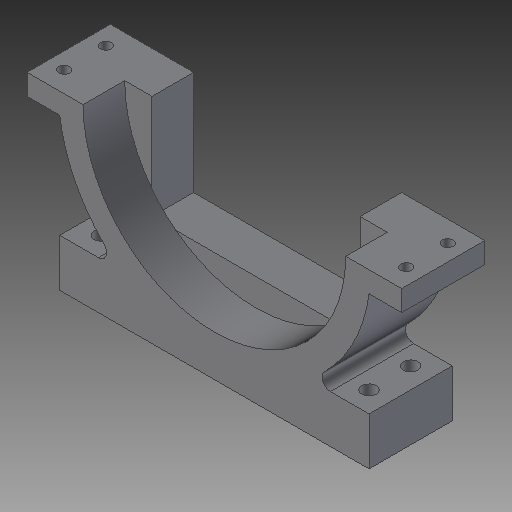
# Autodesk Inventor part: 2124_Bearing Clamps NoPulley_V2
Saved by Autodesk Inventor 2020 (Build 240168000, 168)
## iProperties
Created: 2017-06-21
Part Number: 2124_Bearing Clamps NoPulley_V2
Material: ABS Plastic
Document SubType Name: Modeling
Designer: MPI
Density: 1.06 g/cm^3
Appearance: Smooth - White
Mass: 514.652 g
Surface Area: 684.25 cm^2
Volume: 485.521 cm^3
Author: MPI
Autodesk Inventor part; units mm, degrees
ref_plane "YZ Plane" through (0, 0, 0) normal (1, 0, 0) x (0, 1, 0)
ref_plane "XZ Plane" through (0, 0, 0) normal (0, 1, 0) x (-1, 0, 0)
ref_plane "XY Plane" through (0, 0, 0) normal (0, 0, 1) x (1, 0, 0)
sketch "Sketch1" plane through (0, 0, 0) normal (0, 0, 1) x (1, 0, 0)
  circle A0 centre (0, 0) radius 80.137
  line L0 (-114.3, -12.7) -> (-114.3, 12.7)
  line L1 (114.3, 12.7) -> (114.3, -12.7)
  line L2 (114.3, -12.7) -> (-114.3, 12.7) construction
  line L3 (-114.3, -12.7) -> (114.3, 12.7) construction
  line L4 (-114.3, 0) -> (95.25, 0) construction
  line L5 (-114.3, 12.7) -> (-94.3995, 12.7)
  line L6 (94.3995, 12.7) -> (114.3, 12.7)
  arc A1 (-94.3995, -12.7) -> (94.3995, -12.7) centre (0, 0) ccw
  arc A2 (94.3995, 12.7) -> (-94.3995, 12.7) centre (0, 0) ccw
  line L7 (114.3, -12.7) -> (94.3995, -12.7)
  line L8 (-94.3995, -12.7) -> (-114.3, -12.7)
  dimension "d0" = 160.274
  dimension "d2" = 228.6
  dimension "d3" = 25.4
  constraints: 18 end point, 7 parallel, 4 point on circle, 3 centre point, 3 midpoint, 2 coincident, 2 horizontal, 2 perpendicular
  measures "d0" diameter of A0
  measures "d2" distance of L1.end L0.start
  measures "d3" distance of L0.start L0.end
extrude "Extrusion1" add sketch "Sketch1" along normal blind 25.4
sketch "Sketch2" plane through (94.3995, 12.7, 0) normal (0, 1, 0) x (1, 0, 0)
  line L0 (19.9005, 0) -> (0, 0) projected
  line L1 (0, 0) -> (0, -25.4) projected
  line L2 (19.9005, -25.4) -> (0, -25.4) projected
  line L3 (19.9005, 0) -> (19.9005, -25.4) projected
  line L4 (19.9005, -12.7) -> (0, -12.7) construction
  line L5 (9.9502, -25.4) -> (9.9502, 0) construction
  circle A0 centre (9.9502, -12.7) radius 3.3782
  point P0 (-94.3995, 0)
  dimension "d6" = 6.7564
  constraints: 5 midpoint, 4 end point, 1 centre point
  measures "d6" diameter of A0
extrude "Extrusion2" cut sketch "Sketch2" against normal blind 38.1 contours A0
sketch "Sketch3" plane through (94.3995, 12.7, 0) normal (0, 1, 0) x (1, 0, 0)
  circle A0 centre (9.9502, -12.7) radius 3.175
  line L0 (9.9502, -4.8005) -> (16.7914, -8.7502)
  line L1 (16.7914, -8.7502) -> (16.7914, -16.6498)
  line L2 (16.7914, -16.6498) -> (9.9502, -20.5995)
  line L3 (9.9502, -20.5995) -> (3.1091, -16.6498)
  line L4 (3.1091, -16.6498) -> (3.1091, -8.7502)
  line L5 (3.1091, -8.7502) -> (9.9502, -4.8005)
  point P0 (-94.3995, 0)
  constraints: 12 end point, 1 centre point, 1 coincident, 13 other
extrude "Extrusion3" [suppressed]
mirror "Mirror1" about plane through (0, 0, 0) normal (1, 0, 0) of "Extrusion2"
sketch "Sketch6" plane through (0, 0, 25.4) normal (0, 0, 1) x (1, 0, 0)
  line L0 (-63.5, -63.5) -> (-63.5, 63.5) construction
  line L1 (-63.5, 63.5) -> (63.5, 63.5) construction
  line L2 (63.5, 63.5) -> (63.5, -63.5) construction
  line L3 (63.5, -63.5) -> (-63.5, -63.5) construction
  line L4 (-94.3995, 94.3995) -> (-63.5, 63.5) construction
  line L5 (63.5, 63.5) -> (94.3995, 94.3995) construction
  line L6 (63.5, -63.5) -> (94.3995, -94.3995) construction
  line L7 (-63.5, -63.5) -> (63.5, -63.5) construction
  line L8 (-63.5, -63.5) -> (-94.3995, -94.3995) construction
  point P0 (-78.9498, 78.9498)
  point P1 (78.9498, 78.9498)
  point P2 (78.9498, -78.9498)
  point P3 (-78.9498, -78.9498)
  constraints: 8 end point, 4 midpoint, 3 perpendicular
hole "Hole1" [suppressed]
sketch "Sketch9" plane through (0, 0, 25.4) normal (0, 0, 1) x (1, 0, 0)
  line L0 (114.3, -12.7) -> (114.3, 12.7) projected
  line L1 (114.3, 12.7) -> (94.3995, 12.7) projected
  line L2 (94.3995, 12.7) -> (94.3995, 94.3995) projected
  line L3 (94.3995, 94.3995) -> (12.7, 94.3995) projected
  arc A0 (94.3995, 12.7) -> (-94.3995, 12.7) centre (0, 0) ccw projected
  line L4 (-12.7, 94.3995) -> (-94.3995, 94.3995) projected
  line L5 (-94.3995, 94.3995) -> (-94.3995, 12.7) projected
  line L6 (-94.3995, 12.7) -> (-114.3, 12.7) projected
  line L7 (-114.3, 12.7) -> (-114.3, -12.7) projected
  line L8 (-114.3, 0) -> (114.3, 0)
  constraints: 2 end point, 2 midpoint
extrude "Extrusion7" cut sketch "Sketch9" against normal blind 25.4
sketch "Sketch10" plane through (0, 0, 0) normal (0, 0, -1) x (-1, 0, 0)
  arc A0 (-94.3995, -12.7) -> (94.3995, -12.7) centre (0, 0) ccw projected
  line L0 (-63.5, -63.5) -> (63.5, -63.5)
  line L1 (63.5, -63.5) -> (63.5, 63.5)
  line L2 (63.5, 63.5) -> (-63.5, 63.5)
  line L3 (-63.5, 63.5) -> (-63.5, -63.5)
  line L4 (-63.5, -63.5) -> (63.5, 63.5) construction
  line L5 (63.5, -63.5) -> (-63.5, 63.5) construction
  circle A1 centre (0, 0) radius 95.25
  dimension "d58" = 127
  dimension "d59" = 127
  constraints: 12 end point, 2 midpoint, 2 parallel, 1 centre point, 1 coincident, 1 horizontal, 1 perpendicular
  measures "d58" distance of L2.end L1.end
  measures "d59" distance of L1.end L0.end
extrude "Extrusion8" add sketch "Sketch10" along normal blind 25.4
sketch "Sketch12" plane through (0, 0, 0) normal (0, 0, 1) x (1, 0, 0)
  line L0 (-80.137, 0) -> (-114.3, 0) projected
  line L1 (-114.3, 0) -> (111.125, 0)
  line L2 (111.125, 0) -> (111.125, 104.775)
  line L3 (111.125, 104.775) -> (-114.3, 104.775)
  line L4 (-114.3, 104.775) -> (-114.3, 0)
  point P0 (0, 0)
  point P1 (-83.312, 0)
  constraints: 8 end point, 2 parallel, 1 horizontal, 1 perpendicular
extrude "Extrusion10" cut sketch "Sketch12" against normal blind 25.4
sketch "Sketch14" plane through (0, 0, 25.4) normal (0, 0, 1) x (1, 0, 0)
  line L0 (80.137, 0) -> (63.5, 0) projected
  line L1 (-114.3, -12.7) -> (-94.3995, -12.7) projected
  line L2 (94.3995, -105.25) -> (-94.3995, -105.25)
  line L3 (0, -95.25) -> (-39.6875, -95.25)
  arc A0 (-94.3995, -12.7) -> (94.3995, -12.7) centre (0, 0) ccw
  line L4 (94.3995, -76.2) -> (57.15, -76.2)
  line L5 (-94.3995, -76.2) -> (-57.15, -76.2)
  arc A1 (-57.15, -76.2) -> (57.15, -76.2) centre (0, 0) ccw
  line L6 (94.3995, -105.25) -> (94.3995, -76.2)
  line L7 (-94.3995, -105.25) -> (-94.3995, -76.2)
  point P0 (-80.137, 0)
  dimension "d74" = 10
  constraints: 12 end point, 6 point on circle, 2 centre point, 2 coincident, 2 horizontal, 2 point on line, 1 parallel, 1 vertical
  measures "d74" distance between parallel lines of L2 L3
extrude "Extrusion11" add sketch "Sketch14" against normal up to surface (50.8 mm away)
fillet "Fillet1" radius 5.08 4 edges at (-57.15, -76.2, 12.7) (-57.15, -76.2, -12.7) (57.15, -76.2, 12.7) (57.15, -76.2, -12.7)
sketch "Sketch16" plane through (-94.3995, -105.25, 25.4) normal (0, -1, 0) x (1, 0, 0)
  circle A0 centre (12.7, -38.1) radius 4.5
  line L0 (0, 0) -> (0, -50.8) projected
  line L1 (188.7991, -50.8) -> (0, -50.8) projected
  circle A1 centre (12.7, -12.7) radius 4.5
  line L2 (0, 0) -> (188.7991, 0) projected
  circle A2 centre (176.0991, -38.1) radius 4.5
  circle A3 centre (176.0991, -12.7) radius 4.5
  line L3 (188.7991, 0) -> (188.7991, -50.8) projected
  point P0 (94.3995, -25.4)
  dimension "d76" = 9
  dimension "d77" = 12.7
  dimension "d78" = 12.7
  dimension "d79" = 9
  dimension "d80" = 12.7
  dimension "d81" = 12.7
  dimension "d82" = 9
  dimension "d83" = 9
  dimension "d84" = 12.7
  dimension "d85" = 12.7
  dimension "d88" = 12.7
  dimension "d89" = 12.7
  constraints: 4 centre point
  measures "d76" diameter of A0
  measures "d77" distance from line of L0 A0.centre
  measures "d78" distance from line of L1 A0.centre
  measures "d79" diameter of A1
  measures "d80" distance from line of L0 A1.centre
  measures "d81" distance from line of L2 A1.centre
  measures "d82" diameter of A2
  measures "d83" diameter of A3
  measures "d84" distance from line of L3 A2.centre
  measures "d85" distance from line of L3 A3.centre
  measures "d88" distance from line of L1 A2.centre
  measures "d89" distance from line of L2 A3.centre
extrude "Extrusion12" cut sketch "Sketch16" against normal up to surface (29.05 mm away) contours A0 | A1 | A2 | A3
sketch "Sketch17" plane through (0, 0, 0) normal (0, 0, -1) x (-1, 0, 0)
  arc A0 (-95.25, 0) -> (-94.3995, -12.7) centre (0, 0) ccw projected
  line L0 (-95.25, 0) -> (-114.3, 0) projected
  line L1 (-114.3, -12.7) -> (-114.3, 0) projected
  line L2 (-94.3995, -12.7) -> (-114.3, -12.7) projected
  arc A1 (94.3995, -12.7) -> (95.25, 0) centre (0, 0) ccw projected
  line L3 (114.3, -12.7) -> (94.3995, -12.7) projected
  line L4 (114.3, 0) -> (114.3, -12.7) projected
  line L5 (114.3, 0) -> (95.25, 0) projected
extrude "Extrusion13" add sketch "Sketch17" along normal blind 25.4
sketch "Sketch18" plane through (-114.3, -12.7, 25.4) normal (0, -1, 0) x (1, 0, 0)
  circle A0 centre (9.9502, -12.7) radius 3.3782 projected
  circle A1 centre (9.9502, -38.1) radius 3.3782
  line L0 (0, 0) -> (19.9005, 0) projected
  line L1 (19.9005, -50.8) -> (0, -50.8) projected
  line L2 (0, -50.8) -> (0, 0) projected
  circle A2 centre (218.6498, -12.7) radius 3.3782 projected
  circle A3 centre (218.6498, -38.1) radius 3.3782
  line L3 (228.6, 0) -> (228.6, -50.8) projected
  line L4 (208.6995, 0) -> (228.6, 0) projected
  line L5 (228.6, -50.8) -> (208.6995, -50.8) projected
  point P0 (114.3, -25.4)
  dimension "d92" = 6.7564
  dimension "d93" = 6.7564
  dimension "d94" = 12.7
  dimension "d95" = 12.7
  dimension "d96" = 9.9502
  dimension "d97" = 9.9502
  dimension "d98" = 6.7564
  dimension "d99" = 9.9502
  dimension "d100" = 12.7
  dimension "d101" = 9.9502
  dimension "d102" = 12.7
  dimension "d103" = 6.7564
  constraints: 2 centre point
  measures "d92" diameter of A1
  measures "d93" diameter of A0
  measures "d94" distance from line of L0 A0.centre
  measures "d95" distance from line of L1 A1.centre
  measures "d96" distance from line of L2 A0.centre
  measures "d97" distance from line of L2 A1.centre
  measures "d98" diameter of A2
  measures "d99" distance from line of L3 A2.centre
  measures "d100" distance from line of A2.centre L4
  measures "d101" distance from line of L3 A3.centre
  measures "d102" distance from line of L5 A3.centre
  measures "d103" diameter of A3
extrude "Extrusion14" cut sketch "Sketch18" against normal blind 25.4 contours A1 | A3
equation "\"d36\" = 0.25 * d33"
equation "\"d37\" = d36"
equation "\"d33\" = 9.525"
body "Solid1"
body "Solid2"
